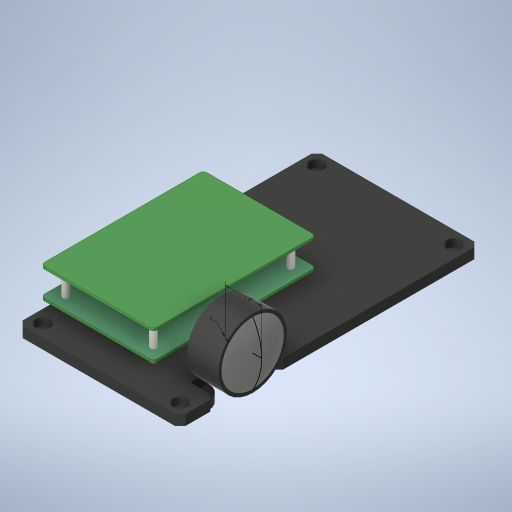
# Autodesk Inventor part: projector1
Saved by Autodesk Inventor 2024 (Build 280153000, 153)
## iProperties
Created: 2018-09-13
Part Number: projector1
Material: Generic
Document SubType Name: Modeling
Designer: Daniel
Density: 1 g/cm^3
Appearance: Smooth - Dark Forest Green
Author: Daniel
Autodesk Inventor part; units mm, degrees
ref_plane "YZ Plane" through (0, 0, 0) normal (1, 0, 0) x (0, 1, 0)
ref_plane "XZ Plane" through (0, 0, 0) normal (0, 1, 0) x (-1, 0, 0)
ref_plane "XY Plane" through (0, 0, 0) normal (0, 0, 1) x (1, 0, 0)
sketch "Sketch1" plane through (0, 0, 0) normal (0, 1, 0) x (-1, 0, 0)
  line L0 (0, 0) -> (129.8, 0)
  line L1 (129.8, 0) -> (129.8, -239)
  line L2 (129.8, -239) -> (0, -239)
  line L3 (0, -239) -> (0, 0)
  line L4 (0, -28) -> (20, -28)
  line L5 (20, -28) -> (20, -78)
  line L6 (20, -78) -> (0, -78)
  line L7 (0, -78) -> (0, -28)
  line L8 (0, -53) -> (20, -53)
  dimension "d0" = 129.8
  dimension "d1" = 239
  dimension "d13" = 20
  dimension "d38" = 53
  dimension "d41" = 28
  dimension "d43" = 50
  constraints: 18 end point, 4 parallel, 3 perpendicular, 2 horizontal, 2 midpoint, 1 point on line
  measures "d0" distance of L1.end L2.end
  measures "d1" distance of L0.end L1.end
  measures "d13" distance of L4.start L4.end
  measures "d38" distance between parallel lines of L0 L8
  measures "d41" distance between parallel lines of L0 L4
  measures "d43" distance between parallel lines of L4 L6
extrude "Extrusion1" add sketch "Sketch1" along normal blind 8.2 contours L0 L1 L2 L3 L6 L5 L4
ref_plane "Work Plane2" through (0, 28.5, 0) normal (0, -1, 0) x (1, 0, 0)
sketch "Sketch4" plane through (0, 28.5, 0) normal (0, -1, 0) x (1, 0, 0)
  line L0 (-20, -80.5) -> (5, -80.5)
  line L1 (5, -80.5) -> (5, -53)
  line L2 (5, -53) -> (-20, -53)
  line L3 (-20, -53) -> (-20, -80.5)
  line L4 (-20, -28) -> (-20, -78) construction
  line L5 (0, 0) -> (0, -28) construction
  arc A0 (5, -78) -> (12, -53) centre (-36.1429, -53) ccw
  line L6 (5, -53) -> (12, -53)
  line L7 (-20, -53) -> (20.7311, -53) construction
  line L8 (0, -78) -> (0, -239) projected
  line L9 (-129.8, 0) -> (0, 0) projected
  dimension "d14" = 27.5
  dimension "d16" = 2.5
  dimension "d17" = 7
  dimension "d18" = 25
  dimension "d53" = 12
  dimension "d54" = 53
  constraints: 10 end point, 3 horizontal, 2 point on circle, 1 centre point, 1 collinear, 1 line through centre, 1 midpoint, 1 parallel, 1 point on line, 1 vertical, 3 other
  measures "d14" distance of L2.end L3.end
  measures "d16" distance of L1.start A0.start
  measures "d17" distance of L1.end L6.end
  measures "d18" distance of L1.end L2.end
  measures "d53" distance from line of L6.end L8
  measures "d54" distance between parallel lines of L9 L2
revolve "Revolution2" add sketch "Sketch4" angle 360 about axis through (-20, 28.5, -53) along (1, 0, 0) separate body contours L6 A0 L1
revolve "Revolution4" add sketch "Sketch4" angle 360 about axis through (-20, 28.5, -53) along (1, 0, 0) bodies 1 contours L3 L2 L1 L0
ref_plane "Work Plane3" through (-5, 15, -53) normal (0, 0, -1) x (-1, 0, 0)
sketch "Sketch13" plane through (70, 0, -82) normal (1, 0, 0) x (0, 0, -1)
  line L0 (-29, 28.5) -> (304.7426, 82.8945) projected
  line L1 (-29, 28.5) -> (-385.7911, 81.9726) projected
  line L2 (-29, 28.5) -> (-397.7764, 519.8945) projected
  line L3 (-29, 28.5) -> (307.5084, 535.5675) projected
  line L4 (36.7658, 39.2187) -> (36.8983, 127.7988)
  line L5 (36.8983, 127.7988) -> (-99.6232, 122.6054)
  line L6 (-99.6232, 122.6054) -> (-99.5325, 39.0708)
  line L7 (36.7658, 39.2187) -> (-99.5325, 39.0708)
  point P0 (-82, 0)
  constraints: 8 end point, 4 point on line, 1 perpendicular
sketch "Sketch6" plane through (-5, 15, -53) normal (0, 0, -1) x (-1, 0, 0)
  arc A0 (-10, 38.5) -> (-10, -11.5) centre (31.1429, 13.5) ccw
  line L0 (12, 13.5) -> (-17, 13.5)
  arc A1 (-10, 38.5) -> (-10, -11.5) centre (31.1429, 13.5) ccw projected
  circle A2 centre (12, 13.5) radius 3.5
  line L1 (12, 13.5) -> (15.5, 13.5)
  point P0 (-5, -15)
  point P1 (8.5, 13.5)
  dimension "d102" = 7
  dimension "d67" = 29
  dimension "d72" = 63.5
  dimension "d73" = 64
  dimension "d74" = 309.5
  dimension "d75" = 301
  dimension "d76" = 193.5
  dimension "d77" = 200
  dimension "d78" = 181
  dimension "d79" = 182.5
  constraints: 8 end point
  measures "d76" horizontal distance of A2.centre L0.end
  measures "d77" horizontal distance of A2.centre L0.start
  measures "d78" horizontal distance of A2.centre L1.end
sketch "Sketch7" plane through (0, 8.2, 0) normal (0, 1, 0) x (1, 0, 0)
  circle A0 centre (-10, 10) radius 3.5
  circle A1 centre (-119.8, 10) radius 3.5
  circle A2 centre (-119.8, 229) radius 3.5
  circle A3 centre (-10, 229) radius 3.5
  line L0 (-129.8, 0) -> (0, 0) projected
  line L1 (-129.8, 239) -> (-129.8, 0) projected
  line L2 (0, 78) -> (0, 239) projected
  line L3 (0, 239) -> (-129.8, 239) projected
  point P0 (-124.8, 0)
  point P1 (-5, 0)
  point P2 (-129.8, 234)
  point P3 (-129.8, 5)
  point P4 (0, 5)
  point P5 (0, 23)
  point P6 (-5, 239)
  point P7 (-124.8, 239)
  dimension "d25" = 7
  dimension "d26" = 7
  dimension "d27" = 7
  dimension "d28" = 7
  dimension "d29" = 10
  dimension "d30" = 10
  dimension "d31" = 10
  dimension "d32" = 10
  constraints: 4 centre point, 2 horizontal alignment, 2 vertical alignment
  measures "d25" diameter of A0
  measures "d26" diameter of A1
  measures "d27" diameter of A2
  measures "d28" diameter of A3
  measures "d29" distance from line of L0 A1.centre
  measures "d30" distance from line of L1 A1.centre
  measures "d31" distance from line of L2 A0.centre
  measures "d32" distance from line of L3 A2.centre
extrude "Extrusion3" cut sketch "Sketch7" against normal through all bodies 1
sketch "Sketch8" plane through (0, 8.2, 0) normal (0, 1, 0) x (1, 0, 0)
  circle A0 centre (-10, 10) radius 3.5 projected
  circle A1 centre (-10, 10) radius 6
  circle A2 centre (-119.8, 10) radius 3.5 projected
  circle A3 centre (-119.8, 10) radius 6
  circle A4 centre (-119.8, 229) radius 3.5 projected
  circle A5 centre (-119.8, 229) radius 6
  circle A6 centre (-10, 229) radius 3.5 projected
  circle A7 centre (-10, 229) radius 6
  point P0 (0, 0)
  dimension "d44" = 12
  dimension "d45" = 12
  dimension "d46" = 12
  dimension "d47" = 12
  constraints: 4 centre point, 4 coincident
  measures "d44" diameter of A5
  measures "d45" diameter of A3
  measures "d46" diameter of A7
  measures "d47" diameter of A1
extrude "Extrusion4" cut sketch "Sketch8" against normal blind 10 contours A0 | A1 | A2 | A3 | A4 | A5 | A6 | A7 bodies 1
revolve "Revolution3" add sketch "Sketch6" angle 360 about axis through (-17, 28.5, -53) along (-1, 0, 0) separate body picked at (9.7006, 13.2208) contours L1 A2 L0
chamfer "Chamfer2" distance 4 angle 45 6 edges at (0, 4.1, 0) (-129.8, 4.1, 0) (0, 4.1, -78) (0, 4.1, -28) (0, 4.1, -239) (-129.8, 4.1, -239)
sketch "Sketch9" plane through (0, 0, 0) normal (0, -1, 0) x (1, 0, 0)
  circle A0 centre (-20, -30) radius 12.5
  circle A1 centre (-20, -209) radius 12.5
  circle A2 centre (-109.8, -209) radius 12.5
  circle A3 centre (-109.8, -30) radius 12.5
  line L0 (-125.8, -239) -> (-4, -239) projected
  line L1 (0, -235) -> (0, -82) projected
  line L2 (-129.8, -4) -> (-129.8, -235) projected
  line L3 (-4, 0) -> (-125.8, 0) projected
  point P0 (0, 0)
  dimension "d58" = 25
  dimension "d59" = 25
  dimension "d60" = 25
  dimension "d61" = 25
  dimension "d62" = 30
  dimension "d63" = 20
  dimension "d64" = 20
  dimension "d65" = 30
  constraints: 4 centre point, 2 horizontal alignment, 2 vertical alignment
  measures "d58" diameter of A0
  measures "d59" diameter of A1
  measures "d60" diameter of A2
  measures "d61" diameter of A3
  measures "d62" distance from line of L0 A1.centre
  measures "d63" distance from line of L1 A1.centre
  measures "d64" distance from line of L2 A2.centre
  measures "d65" distance from line of L3 A3.centre
extrude "Extrusion5" add sketch "Sketch9" along normal blind 6 bodies 1
sketch "Sketch14" plane through (0, 8.2, 0) normal (0, 1, 0) x (1, 0, 0)
  circle A0 centre (-119.5374, 28) radius 2.5
  circle A1 centre (-119.5374, 138) radius 2.5
  circle A2 centre (-49.5374, 28) radius 2.5
  circle A3 centre (-49.5374, 138) radius 2.5
  circle A4 centre (-119.8, 10) radius 6 projected
  point P0 (0, 0)
  dimension "d103" = 5
  dimension "d104" = 110
  dimension "d105" = 70
  dimension "d106" = 18
  constraints: 4 centre point, 3 equal radius, 2 horizontal alignment, 2 vertical alignment
  measures "d103" diameter of A0
  measures "d104" distance of A1.centre A0.centre
  measures "d105" distance of A1.centre A3.centre
  measures "d106" vertical distance of A4.centre A0.centre
extrude "Extrusion7" add sketch "Sketch14" along normal blind 30 separate body contours A0 | A1 | A2 | A3
sketch "Sketch15" plane through (-119.5374, 38.2, -28) normal (0, 1, 0) x (1, 0, 0)
  circle A0 centre (0, 0) radius 2.5 construction
  circle A1 centre (70, 110) radius 2.5 construction
  line L0 (0, 0) -> (70, 0)
  line L1 (70, 0) -> (70, 110) construction
  line L2 (70, 110) -> (0, 110)
  line L3 (0, 110) -> (0, 0)
  line L4 (80, 117) -> (80, -7)
  line L5 (77, -10) -> (-7, -10)
  line L6 (-10, -7) -> (-10, 117)
  line L7 (-7, 120) -> (77, 120)
  arc A2 (77, -10) -> (80, -7) centre (77, -7) ccw
  arc A3 (-10, -7) -> (-7, -10) centre (-7, -7) ccw
  arc A4 (-7, 120) -> (-10, 117) centre (-7, 117) ccw
  arc A5 (80, 117) -> (77, 120) centre (77, 117) ccw
  point P0 (119.5374, -28)
  dimension "d110" = 3
  dimension "d111" = 10
  constraints: 16 end point, 8 point on circle, 8 tangent, 4 centre point, 4 parallel, 3 equal radius, 2 perpendicular, 1 horizontal, 3 other
  measures "d110" radius of A2
  measures "d111" distance between parallel lines of L1 L4
extrude "Extrusion8" add sketch "Sketch15" along normal blind 2 separate body
ref_plane "Work Plane9" through (-119.5374, 28.2, -28) normal (0, -1, 0) x (1, 0, 0)
mirror "Mirror1" about plane through (-119.5374, 28.2, -28) normal (0, -1, 0) of "Extrusion8" bodies 5
sketch "Sketch16" plane through (0, 0, 0) normal (0, -1, 0) x (1, 0, 0)
  circle A0 centre (-119.8, -229) radius 6 projected
  circle A1 centre (-10, -229) radius 6 projected
  circle A2 centre (-10, -10) radius 6 projected
  circle A3 centre (-119.8, -10) radius 6 projected
  circle A4 centre (-119.8, -229) radius 3.05
  circle A5 centre (-10, -229) radius 3.05
  circle A6 centre (-10, -10) radius 3.05
  circle A7 centre (-119.8, -10) radius 3.05
  point P0 (0, 0)
  dimension "d115" = 6.1
  dimension "d116" = 6.1
  dimension "d117" = 6.1
  dimension "d118" = 6.1
  constraints: 4 centre point, 4 coincident
  measures "d115" diameter of A4
  measures "d116" diameter of A5
  measures "d117" diameter of A6
  measures "d118" diameter of A7
extrude "Extrusion9" add sketch "Sketch16" against normal blind 2 bodies 1
sketch "Sketch12" plane through (420, 0, -82) normal (1, 0, 0) x (0, 0, -1)
  line L0 (-397.7764, 519.8945) -> (-385.7911, 81.9726)
  line L1 (-385.7911, 81.9726) -> (304.7426, 82.8945)
  line L2 (304.7426, 82.8945) -> (307.5084, 535.5675)
  line L3 (307.5084, 535.5675) -> (-397.7764, 519.8945)
  point P0 (-82, 0)
  constraints: 8 end point
equation "\"d38\" = lensFromRightEdge"
equation "\"d53\" = lensDistance"
equation "\"d62\" = d65"
equation "\"d63\" = d64"
equation "\"d19\" = -lensHeight"
equation "\"lensFromRightEdge\" = 53"
equation "\"lensHeight\" = 28.5"
equation "\"lensDistance\" = 12"
body "Solid4"
